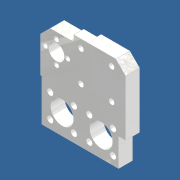
# Autodesk Inventor part: 0008-10-001
Saved by Autodesk Inventor 2020 (Build 240168000, 168)
## iProperties
Created: 2021-02-20
Part Number: 0008-10-001
Material: ABS Plastic
Document SubType Name: Modeling
Designer: Iulian Bors
Density: 1.06 g/cm^3
Appearance: Smooth - White
Mass: 61.7773 g
Surface Area: 186.476 cm^2
Volume: 58.2805 cm^3
Description: Actionator seringa
Sheet Metal Rule: Default
Author: Iulian Bors
Subject: 001
Autodesk Inventor part; units mm, degrees
ref_plane "YZ Plane" through (0, 0, 0) normal (1, 0, 0) x (0, 1, 0)
ref_plane "XZ Plane" through (0, 0, 0) normal (0, 1, 0) x (-1, 0, 0)
ref_plane "XY Plane" through (0, 0, 0) normal (0, 0, 1) x (1, 0, 0)
sketch "Sketch1" plane through (0, 0, 0) normal (0, 0, 1) x (1, 0, 0)
  line L0 (-32.5, 33.5) -> (32.5, 33.5)
  line L1 (32.5, 33.5) -> (32.5, -33.5)
  line L2 (32.5, -33.5) -> (-32.5, -33.5)
  line L3 (-32.5, -33.5) -> (-32.5, 33.5)
  point P0 (0, 0)
  point P1 (0, 33.5)
  point P2 (-32.5, 0)
  dimension "d0" = 65
  dimension "d1" = 67
  constraints: 8 end point, 2 midpoint, 2 parallel, 1 horizontal, 1 horizontal alignment, 1 perpendicular, 1 vertical alignment
  measures "d0" distance of L0.start L0.end
  measures "d1" distance of L0.end L1.end
extrude "Extrusion1" add sketch "Sketch1" along normal blind 10
sketch "Sketch5" plane through (0, 0, 0) normal (0, 0, -1) x (-1, 0, 0)
  circle A0 centre (-0.5, 27.5) radius 2
  circle A1 centre (-0.5, 5.5) radius 2
  line L0 (32.5, 33.5) -> (32.5, -33.5) projected
  line L1 (-32.5, 33.5) -> (32.5, 33.5) projected
  circle A2 centre (-22.5, 5.5) radius 2
  circle A3 centre (-22.5, 27.5) radius 2
  line L2 (-32.5, -33.5) -> (-32.5, 33.5) projected
  point P0 (0, 0)
  dimension "d30" = 6
  dimension "d31" = 4
  dimension "d32" = 22
  dimension "d50" = 22
  dimension "d51" = 10
  constraints: 4 centre point, 3 equal radius, 2 horizontal alignment, 2 vertical alignment
  measures "d30" distance from line of L1 A0.centre
  measures "d31" diameter of A0
  measures "d32" distance of A0.centre A1.centre
  measures "d50" distance of A3.centre A0.centre
  measures "d51" distance from line of L2 A3.centre
hole "Hole1" at (0.5, 5.5, 0) at (0.5, 27.5, 0) at (22.5, 5.5, 0) at (22.5, 27.5, 0) direction (0, 0, 1) diameter 4 depth 11 tip angle 118 counterbore diameter 9 counterbore depth 3
sketch "Sketch6" plane through (0, 0, 0) normal (0, 0, -1) x (-1, 0, 0)
  line L0 (4, 23) -> (-5, 23)
  line L1 (-5, 23) -> (-5, 33.5)
  line L2 (-5, 33.5) -> (4, 33.5)
  line L3 (4, 33.5) -> (4, 23)
  line L4 (-32.5, 33.5) -> (32.5, 33.5) projected
  circle A0 centre (-0.5, 27.5) radius 4.5 projected
  line L5 (6, 29) -> (4, 29)
  line L6 (4, 29) -> (4, 33.5)
  line L7 (4, 33.5) -> (6, 33.5)
  line L8 (6, 33.5) -> (6, 29)
  point P0 (0, 0)
  point P1 (-5, 27.5)
  point P2 (4, 27.5)
  point P3 (6, 33.5)
  point P4 (4, 33.5)
  point P5 (4, 29)
  dimension "d77" = 2
  dimension "d78" = 4.5
  constraints: 16 end point, 4 parallel, 3 collinear, 3 tangent, 2 horizontal, 2 perpendicular
  measures "d77" distance of L5.start L5.end
  measures "d78" distance between parallel lines of L4 L5
extrude "Extrusion4" cut sketch "Sketch6" against normal up to surface (3 mm away) contours A0 L1 L2 L3 | L3 L4 L8 L5
sketch "Sketch7" plane through (0, 0, 0) normal (0, 0, -1) x (-1, 0, 0)
  circle A0 centre (17, 16.5) radius 5.75
  circle A1 centre (17, 16.5) radius 8 construction
  circle A2 centre (17, 24.5) radius 1.75
  line L0 (6, 33.5) -> (32.5, 33.5) projected
  line L1 (32.5, 33.5) -> (32.5, -33.5) projected
  circle A3 centre (9, 16.5) radius 1.75
  circle A4 centre (17, 8.5) radius 1.75
  circle A5 centre (25, 16.5) radius 1.75
  line L2 (6, 33.5) -> (-5, 33.5) projected
  line L3 (-32.5, -33.5) -> (-32.5, 33.5) projected
  point P0 (4, 33.5)
  point P1 (25.5, 33.5)
  point P2 (32.5, 26.5)
  point P3 (-25.5, 33.5)
  point P4 (-32.5, 26.5)
  dimension "d55" = 16
  dimension "d52" = 11.5
  dimension "d54" = 3.5
  dimension "d61" = 360
  dimension "d65" = 17
  dimension "d66" = 49.5
  constraints: 5 centre point, 2 vertical alignment, 1 coincident, 11 other
  measures "d52" diameter of A0
  measures "d54" diameter of A2
  measures "d65" distance from line of L2 A0.centre
  measures "d66" distance from line of L3 A0.centre
extrude "Extrusion5" cut sketch "Sketch7" against normal through all
sketch "Sketch8" plane through (0, 0, 0) normal (0, 0, -1) x (-1, 0, 0)
  line L0 (32.5, -33.5) -> (-32.5, -33.5) projected
  line L1 (32.5, -33.5) -> (27.5, -33.5)
  line L2 (27.5, -33.5) -> (27.5, -3.5)
  line L3 (27.5, -3.5) -> (32.5, -3.5)
  line L4 (32.5, -3.5) -> (32.5, -33.5)
  line L5 (-27.5, -33.5) -> (-32.5, -33.5)
  line L6 (-32.5, -33.5) -> (-32.5, -13.5)
  line L7 (-32.5, -13.5) -> (-27.5, -13.5)
  line L8 (-27.5, -13.5) -> (-27.5, -33.5)
  line L9 (32.5, -33.5) -> (-32.5, -33.5) projected
  line L10 (-32.5, -33.5) -> (-32.5, 33.5) projected
  line L11 (32.5, 33.5) -> (32.5, -33.5) projected
  point P0 (0, 0)
  point P1 (-32.5, 26.5)
  point P2 (32.5, 26.5)
  dimension "d67" = 5
  dimension "d68" = 5
  dimension "d69" = 30
  dimension "d72" = 20
  constraints: 16 end point, 4 parallel, 3 collinear, 2 horizontal, 2 perpendicular, 1 point on line
  measures "d67" distance of L2.end L3.end
  measures "d68" distance of L6.end L7.end
  measures "d69" distance of L1.end L2.end
  measures "d72" distance of L7.end L5.start
extrude "Extrusion6" cut sketch "Sketch8" against normal through all
sketch "Sketch9" plane through (0, 0, 10) normal (0, 0, 1) x (1, 0, 0)
  line L0 (-30.5, 33) -> (-7.5, 33)
  line L1 (-32.5, 33.5) -> (-4.5, 33.5)
  line L2 (-4.5, 33.5) -> (-4.5, 29)
  line L3 (-4.5, 29) -> (-32.5, 29)
  line L4 (-32.5, 29) -> (-32.5, 33.5)
  line L5 (-32.5, 33.5) -> (-32.5, -3.5) projected
  line L6 (32.5, 33.5) -> (-32.5, 33.5) projected
  point P0 (0, 0)
  point P1 (-32.5, 26.5)
  point P2 (25.5, 33.5)
  point P3 (-25.5, 33.5)
  dimension "d73" = 4
  dimension "d74" = 3
  constraints: 10 end point, 2 collinear, 2 horizontal, 2 parallel, 1 perpendicular, 2 other
  measures "d73" distance between parallel lines of L3 L0
  measures "d74" distance from line of L2 L0.end
extrude "Extrusion7" cut sketch "Sketch9" against normal through all
sketch "Sketch10" plane through (0, 0, 0) normal (0, 0, -1) x (-1, 0, 0)
  circle A0 centre (-15, -19) radius 4
  circle A1 centre (-23.4853, -10.5147) radius 1.7
  circle A2 centre (-6.5147, -10.5147) radius 1.7
  circle A3 centre (-6.5147, -27.4853) radius 1.7
  circle A4 centre (-23.4853, -27.4853) radius 1.7
  circle A5 centre (-15, -19) radius 7.5
  line L0 (-25.1274, -6.5) -> (-4.8726, -6.5)
  line L1 (-4.8726, -6.5) -> (-2.5, -8.8726)
  line L2 (-2.5, -8.8726) -> (-2.5, -29.1274)
  line L3 (-2.5, -29.1274) -> (-4.8726, -31.5)
  line L4 (-4.8726, -31.5) -> (-25.1274, -31.5)
  line L5 (-25.1274, -31.5) -> (-27.5, -29.1274)
  line L6 (-27.5, -29.1274) -> (-27.5, -8.8726)
  line L7 (-27.5, -8.8726) -> (-25.1274, -6.5)
  circle A6 centre (13, -19) radius 4
  circle A7 centre (21.4853, -10.5147) radius 1.7
  circle A8 centre (21.4853, -27.4853) radius 1.7
  circle A9 centre (4.5147, -27.4853) radius 1.7
  circle A10 centre (4.5147, -10.5147) radius 1.7
  circle A11 centre (13, -19) radius 7.5
  line L8 (25.5, -8.8726) -> (25.5, -29.1274)
  line L9 (25.5, -29.1274) -> (23.1274, -31.5)
  line L10 (23.1274, -31.5) -> (2.8726, -31.5)
  line L11 (2.8726, -31.5) -> (0.5, -29.1274)
  line L12 (0.5, -29.1274) -> (0.5, -8.8726)
  line L13 (0.5, -8.8726) -> (2.8726, -6.5)
  line L14 (2.8726, -6.5) -> (23.1274, -6.5)
  line L15 (23.1274, -6.5) -> (25.5, -8.8726)
  circle A12 centre (-15, -19) radius 8.25
  circle A13 centre (13, -19) radius 8.25
  circle A14 centre (21.4853, -27.4853) radius 2.25
  circle A15 centre (4.5147, -27.4853) radius 2.25
  circle A16 centre (21.4853, -10.5147) radius 2.25
  circle A17 centre (4.5147, -10.5147) radius 2.25
  circle A18 centre (-6.5147, -27.4853) radius 2.25
  circle A19 centre (-23.4853, -27.4853) radius 2.25
  circle A20 centre (-23.4853, -10.5147) radius 2.25
  circle A21 centre (-6.5147, -10.5147) radius 2.25
  point P0 (0, 0)
  dimension "d79" = 16.5
  dimension "d80" = 16.5
  dimension "d81" = 4.5
  dimension "d82" = 4.5
  dimension "d83" = 4.5
  dimension "d84" = 4.5
  dimension "d85" = 4.5
  dimension "d86" = 4.5
  dimension "d87" = 4.5
  dimension "d88" = 4.5
  constraints: 32 end point, 22 centre point, 10 coincident, 4 horizontal, 4 vertical, 48 other
  measures "d79" diameter of A12
  measures "d80" diameter of A13
  measures "d81" diameter of A14
  measures "d82" diameter of A15
  measures "d83" diameter of A16
  measures "d84" diameter of A17
  measures "d85" diameter of A18
  measures "d86" diameter of A19
  measures "d87" diameter of A20
  measures "d88" diameter of A21
extrude "Extrusion8" cut sketch "Sketch10" against normal through all contours A0 | A1 | A2 | A3 | A4 | A5 | A6 | A7 | A8 | A9 | A10 | A11 | A12 | A13 | A14 | A15 | A16 | A17 | A18 | A19 | A20 | A21
move faces "Move1" translate (4, 0, 0) faces at (-32.5, 18.1667, 3.3333)
chamfer "Chamfer2" distance 7 angle 45 2 edges at (-28.5, 29, 5) (32.5, 33.5, 5)
fillet "Fillet1" radius 2 1 edges at (-4.5, 29, 6.5)
equation "\"d50\" = d32"
equation "\"d68\" = d67"
equation "\"d80\" = d79"
equation "\"BendRadius\" = Thickness"
equation "\"BendReliefWidth\" = Thickness"
equation "\"BendReliefDepth\" = 0.5 * Thickness"
equation "\"CornerReliefSize\" = 4 * Thickness"
equation "\"MinimumRemnant\" = 2 * Thickness"
equation "\"TransitionRadius\" = BendRadius"
equation "\"JacobiRadiusSize\" = Thickness"
equation "\"GapSize\" = Thickness"
equation "\"Thickness\" = 0.5"
body "Solid1"
